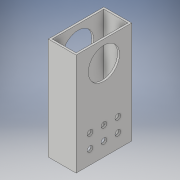
# Autodesk Inventor part: anchor point
Saved by Autodesk Inventor 2018 (Build 220112000, 112)
## iProperties
Created: 2020-01-25
Part Number: anchor point
Material: Generic
Document SubType Name: Modeling
Designer: s-2513225
Density: 1 g/cm^3
Appearance: Default
Author: s-2513225
Autodesk Inventor part; units mm, degrees
ref_plane "YZ Plane" through (0, 0, 0) normal (1, 0, 0) x (0, 1, 0)
ref_plane "XZ Plane" through (0, 0, 0) normal (0, 1, 0) x (-1, 0, 0)
ref_plane "XY Plane" through (0, 0, 0) normal (0, 0, 1) x (1, 0, 0)
sketch "Sketch2" plane through (0, 0, 0) normal (0, 1, 0) x (-1, 0, 0)
  line L0 (0, 0) -> (-25.4, 0)
  line L1 (-25.4, 0) -> (-25.4, -50.8)
  line L2 (-25.4, -50.8) -> (0, -50.8)
  line L3 (0, -50.8) -> (0, 0)
  line L4 (-1.778, -1.778) -> (-23.622, -1.778)
  line L5 (-23.622, -1.778) -> (-23.622, -49.022)
  line L6 (-23.622, -49.022) -> (-1.778, -49.022)
  line L7 (-1.778, -49.022) -> (-1.778, -1.778)
  dimension "d0" = 25.4
  dimension "d1" = 50.8
  dimension "d2" = 1.778
  constraints: 16 end point, 4 parallel, 2 perpendicular, 1 horizontal, 3 other
  measures "d0" distance of L2.end L1.end
  measures "d1" distance of L1.end L0.end
  measures "d2" distance between parallel lines of L3 L7
extrude "Extrusion1" add sketch "Sketch2" along normal blind 93.345
sketch "Sketch3" plane through (25.4, 0, 0) normal (1, 0, 0) x (0, 0, -1)
  line L0 (1.778, 0) -> (49.022, 0) construction
  line L1 (25.4, 0) -> (25.4, 48.768) construction
  line L2 (25.4, 48.768) -> (25.4, 74.168) construction
  circle A0 centre (25.4, 74.168) radius 14.2875
  point P0 (0, 0)
  dimension "d5" = 48.768
  dimension "d6" = 25.4
  dimension "d7" = 28.575
  constraints: 4 end point, 2 vertical, 1 centre point, 1 coincident, 1 midpoint
  measures "d5" distance of L1.start L1.end
  measures "d6" distance of L1.end L2.end
  measures "d7" diameter of A0
extrude "Extrusion2" cut sketch "Sketch3" against normal blind 42.545
sketch "Sketch4" plane through (25.4, 0, 0) normal (1, 0, 0) x (0, 0, -1)
  line L0 (0, 0) -> (12.7, 0) construction
  line L1 (50.8, 0) -> (0, 0) construction
  line L2 (12.7, 0) -> (25.4, 0) construction
  line L3 (25.4, 0) -> (38.1, 0) construction
  line L4 (12.7, 0) -> (12.7, 12.7) construction
  line L5 (12.7, 12.7) -> (12.7, 25.4) construction
  circle A0 centre (12.7, 25.4) radius 2.5797
  circle A1 centre (12.7, 12.7) radius 2.5797
  line L6 (12.7, 25.4) -> (25.4, 25.4) construction
  line L7 (25.4, 25.4) -> (38.1, 25.4) construction
  line L8 (25.4, 12.7) -> (25.4, 25.4) construction
  circle A2 centre (25.4, 25.4) radius 2.5797
  circle A3 centre (25.4, 12.7) radius 2.5797
  line L9 (38.1, 12.7) -> (38.1, 25.4) construction
  circle A4 centre (38.1, 25.4) radius 2.5797
  circle A5 centre (38.1, 12.7) radius 2.5797
  dimension "d10" = 12.7
  dimension "d11" = 12.7
  dimension "d12" = 12.7
  dimension "d13" = 12.7
  dimension "d14" = 12.7
  dimension "d15" = 5.1594
  dimension "d16" = 5.1594
  dimension "d17" = 12.7
  dimension "d27" = 12.7
  dimension "d28" = 12.7
  dimension "d29" = 5.1594
  dimension "d30" = 5.1594
  dimension "d31" = 12.7
  dimension "d32" = 5.1594
  dimension "d33" = 5.1594
  constraints: 18 end point, 6 centre point, 6 coincident, 3 vertical, 2 horizontal, 2 point on line, 1 midpoint, 1 perpendicular
  measures "d10" distance of L0.start L0.end
  measures "d11" distance of L0.end L2.end
  measures "d12" distance of L2.end L3.end
  measures "d13" distance of L0.end L4.end
  measures "d14" distance of L4.end L5.end
  measures "d15" diameter of A0
  measures "d16" diameter of A1
  measures "d17" distance of L6.start L6.end
  measures "d27" distance of L6.end L7.end
  measures "d28" distance of L8.start L8.end
  measures "d29" diameter of A2
  measures "d30" diameter of A3
  measures "d31" distance of L9.start L9.end
  measures "d32" diameter of A4
  measures "d33" diameter of A5
extrude "Extrusion3" cut sketch "Sketch4" against normal blind 25.4
body "Solid1"
